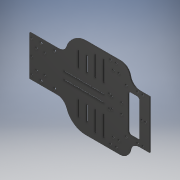
# Autodesk Inventor part: Base
Saved by Autodesk Inventor 2019 (Build 230136000, 136)
## iProperties
Created: 2019-07-29
Part Number: Base
Material: Résine phénolique
Document SubType Name: Modeling
Designer: Sébastien DI MERCURIO
Mass: 119.758 g
Surface Area: 806.74 cm^2
Volume: 86.7812 cm^3
Density: 1.38 g/cm^3
Appearance: Lisse - Noir
Author: Sébastien DI MERCURIO
Autodesk Inventor part; units mm, degrees
ref_plane "YZ Plane" through (0, 0, 0) normal (1, 0, 0) x (0, 1, 0)
ref_plane "XZ Plane" through (0, 0, 0) normal (0, 1, 0) x (-1, 0, 0)
ref_plane "XY Plane" through (0, 0, 0) normal (0, 0, 1) x (1, 0, 0)
sketch "Esquisse1" plane through (0, 0, 0) normal (0, 0, 1) x (1, 0, 0)
  line L0 (-242, 163) -> (0, 163)
  line L1 (0, 163) -> (0, 0)
  line L2 (0, 0) -> (-242, 0)
  line L3 (-242, 0) -> (-242, 163)
  dimension "d0" = 242
  dimension "d1" = 163
  constraints: 8 end point, 2 parallel, 1 horizontal, 1 perpendicular
  measures "d0" distance of L0.start L0.end
  measures "d1" distance of L0.end L1.end
extrude "Extrusion1" add sketch "Esquisse1" along normal blind 2.2
sketch "Esquisse2" plane through (0, 0, 2.2) normal (0, 0, 1) x (1, 0, 0)
  line L0 (0, 0) -> (-40, 0)
  line L1 (-40, 0) -> (-40, 33)
  line L2 (-40, 33) -> (0, 33)
  line L3 (0, 33) -> (0, 0)
  line L4 (0, 163) -> (-242, 163) projected
  line L5 (0, 163) -> (-40, 163)
  line L6 (-40, 163) -> (-40, 130)
  line L7 (-40, 130) -> (0, 130)
  line L8 (0, 130) -> (0, 163)
  line L9 (-242, 163) -> (-166, 163)
  line L10 (-166, 163) -> (-166, 121.5)
  line L11 (-166, 121.5) -> (-242, 121.5)
  line L12 (-242, 121.5) -> (-242, 163)
  line L13 (-242, 0) -> (-166, 0)
  line L14 (-166, 0) -> (-166, 41.5)
  line L15 (-166, 41.5) -> (-242, 41.5)
  line L16 (-242, 41.5) -> (-242, 0)
  dimension "d4" = 97
  dimension "d5" = 80
  dimension "d6" = 76
  dimension "d7" = 40
  constraints: 32 end point, 8 parallel, 4 horizontal, 4 perpendicular, 4 point on line, 2 collinear
  measures "d4" distance of L2.end L7.end
  measures "d5" distance between parallel lines of L15 L11
  measures "d6" distance of L14.end L15.end
  measures "d7" distance of L1.end L2.end
extrude "Extrusion2" cut sketch "Esquisse2" against normal through all
sketch "Esquisse3" plane through (0, 0, 2.2) normal (0, 0, 1) x (1, 0, 0)
  line L0 (-43, 119.5) -> (-20, 119.5)
  line L1 (-20, 119.5) -> (-20, 43.5)
  line L2 (-20, 43.5) -> (-43, 43.5)
  line L3 (-43, 43.5) -> (-43, 119.5)
  line L4 (0, 33) -> (0, 130) projected
  line L5 (0, 130) -> (-40, 130) projected
  line L6 (-92, 149.5) -> (-92, 109.5) construction
  line L7 (-93.5, 149.5) -> (-93.5, 109.5)
  line L8 (-90.5, 109.5) -> (-90.5, 149.5)
  arc A0 (-90.5, 149.5) -> (-93.5, 149.5) centre (-92, 149.5) ccw
  arc A1 (-93.5, 109.5) -> (-90.5, 109.5) centre (-92, 109.5) ccw
  line L9 (-109, 149.5) -> (-109, 109.5) construction
  line L10 (-110.5, 149.5) -> (-110.5, 109.5)
  line L11 (-107.5, 109.5) -> (-107.5, 149.5)
  arc A2 (-107.5, 149.5) -> (-110.5, 149.5) centre (-109, 149.5) ccw
  arc A3 (-110.5, 109.5) -> (-107.5, 109.5) centre (-109, 109.5) ccw
  line L12 (-126, 139.5) -> (-126, 109.5) construction
  line L13 (-127.5, 139.5) -> (-127.5, 109.5)
  line L14 (-124.5, 109.5) -> (-124.5, 139.5)
  arc A4 (-124.5, 139.5) -> (-127.5, 139.5) centre (-126, 139.5) ccw
  arc A5 (-127.5, 109.5) -> (-124.5, 109.5) centre (-126, 109.5) ccw
  line L15 (-143, 139.5) -> (-143, 109.5) construction
  line L16 (-144.5, 139.5) -> (-144.5, 109.5)
  line L17 (-141.5, 109.5) -> (-141.5, 139.5)
  arc A6 (-141.5, 139.5) -> (-144.5, 139.5) centre (-143, 139.5) ccw
  arc A7 (-144.5, 109.5) -> (-141.5, 109.5) centre (-143, 109.5) ccw
  line L18 (-172, 89) -> (-92, 89) construction
  line L19 (-172, 90.5) -> (-92, 90.5)
  line L20 (-92, 87.5) -> (-172, 87.5)
  arc A8 (-172, 90.5) -> (-172, 87.5) centre (-172, 89) ccw
  arc A9 (-92, 87.5) -> (-92, 90.5) centre (-92, 89) ccw
  line L21 (-172, 74) -> (-92, 74) construction
  line L22 (-172, 72.5) -> (-92, 72.5)
  line L23 (-92, 75.5) -> (-172, 75.5)
  arc A10 (-172, 75.5) -> (-172, 72.5) centre (-172, 74) ccw
  arc A11 (-92, 72.5) -> (-92, 75.5) centre (-92, 74) ccw
  line L24 (-92, 53.5) -> (-92, 13.5) construction
  line L25 (-93.5, 53.5) -> (-93.5, 13.5)
  line L26 (-90.5, 13.5) -> (-90.5, 53.5)
  arc A12 (-90.5, 53.5) -> (-93.5, 53.5) centre (-92, 53.5) ccw
  arc A13 (-93.5, 13.5) -> (-90.5, 13.5) centre (-92, 13.5) ccw
  line L27 (-109, 53.5) -> (-109, 13.5) construction
  line L28 (-110.5, 53.5) -> (-110.5, 13.5)
  line L29 (-107.5, 13.5) -> (-107.5, 53.5)
  arc A14 (-107.5, 53.5) -> (-110.5, 53.5) centre (-109, 53.5) ccw
  arc A15 (-110.5, 13.5) -> (-107.5, 13.5) centre (-109, 13.5) ccw
  line L30 (-126, 53.5) -> (-126, 23.5) construction
  line L31 (-127.5, 53.5) -> (-127.5, 23.5)
  line L32 (-124.5, 23.5) -> (-124.5, 53.5)
  arc A16 (-124.5, 53.5) -> (-127.5, 53.5) centre (-126, 53.5) ccw
  arc A17 (-127.5, 23.5) -> (-124.5, 23.5) centre (-126, 23.5) ccw
  line L33 (-143, 53.5) -> (-143, 23.5) construction
  line L34 (-144.5, 53.5) -> (-144.5, 23.5)
  line L35 (-141.5, 23.5) -> (-141.5, 53.5)
  arc A18 (-141.5, 53.5) -> (-144.5, 53.5) centre (-143, 53.5) ccw
  arc A19 (-144.5, 23.5) -> (-141.5, 23.5) centre (-143, 23.5) ccw
  line L36 (-246.6033, 81.5) -> (11.7947, 81.5)
  point P0 (0, 0)
  point P1 (-92, 129.5)
  point P2 (-109, 129.5)
  point P3 (-126, 124.5)
  point P4 (-143, 124.5)
  point P5 (-132, 89)
  point P6 (-132, 74)
  point P7 (-92, 33.5)
  point P8 (-109, 33.5)
  point P9 (-126, 38.5)
  point P10 (-143, 38.5)
  point P11 (-90.5, 89)
  dimension "d10" = 23
  dimension "d11" = 76
  dimension "d12" = 20
  dimension "d14" = 97
  dimension "d15" = 10.5
  dimension "d16" = 3
  dimension "d17" = 3
  dimension "d18" = 3
  dimension "d19" = 3
  dimension "d20" = 3
  dimension "d21" = 3
  dimension "d22" = 3
  dimension "d23" = 3
  dimension "d24" = 3
  dimension "d25" = 3
  dimension "d26" = 12
  dimension "d27" = 14
  dimension "d28" = 14
  dimension "d29" = 14
  dimension "d30" = 33
  dimension "d32" = 43
  dimension "d33" = 80
  dimension "d34" = 92
  dimension "d35" = 48.5
  dimension "d36" = 6
  dimension "d37" = 19
  dimension "d38" = 19
  constraints: 90 end point, 41 point on circle, 40 tangent, 20 centre point, 17 parallel, 10 midpoint, 8 point on line, 7 equal length, 6 horizontal alignment, 2 horizontal, 2 perpendicular, 2 vertical alignment, 1 vertical
  measures "d10" distance of L1.end L2.end
  measures "d11" distance of L0.end L1.end
  measures "d12" distance between parallel lines of L4 L1
  measures "d14" distance of L4.start L4.end
  measures "d15" distance between parallel lines of L0 L5
  measures "d16" distance between parallel lines of L17 L16
  measures "d17" distance between parallel lines of L35 L34
  measures "d18" distance between parallel lines of L32 L31
  measures "d19" distance between parallel lines of L14 L13
  measures "d20" distance between parallel lines of L11 L10
  measures "d21" distance between parallel lines of L8 L7
  measures "d22" distance between parallel lines of L29 L28
  measures "d23" distance between parallel lines of L26 L25
  measures "d24" distance between parallel lines of L20 L19
  measures "d25" distance between parallel lines of L22 L23
  measures "d26" distance between parallel lines of L23 L20
  measures "d27" distance between parallel lines of L7 L11
  measures "d28" distance between parallel lines of L10 L14
  measures "d29" distance between parallel lines of L13 L17
  measures "d33" distance of L18.end L18.start
  measures "d34" distance from line of L18.end L4
  measures "d35" distance between parallel lines of L5 L36
  measures "d36" distance between parallel lines of L36 L20
  measures "d37" distance from line of L19 L6.end
  measures "d38" distance from line of L22 L24.start
extrude "Extrusion3" cut sketch "Esquisse3" against normal through all
sketch "Esquisse4" plane through (0, 0, 2.2) normal (0, 0, 1) x (1, 0, 0)
  line L0 (-257.905, 81.5) -> (33.7686, 81.5)
  line L1 (-40, 33) -> (0, 33) construction
  line L2 (0, 130) -> (-40, 130) construction
  circle A0 centre (-15, 81.5) radius 1.5
  circle A1 centre (-8, 81.5) radius 1.5
  circle A2 centre (-13, 126.5) radius 1.5
  circle A3 centre (-24, 126.5) radius 1.5
  circle A4 centre (-47, 126.5) radius 1.5
  circle A5 centre (-67, 155) radius 1.5
  circle A6 centre (-78.5, 155) radius 1.5
  circle A7 centre (-73, 140) radius 1.5
  circle A8 centre (-61.5, 140) radius 1.5
  circle A9 centre (-56, 91.5) radius 1.5
  circle A10 centre (-76, 92.5) radius 1.5
  circle A11 centre (-81, 94.5) radius 1.5
  circle A12 centre (-228, 101) radius 1.5
  circle A13 centre (-211, 101) radius 1.5
  circle A14 centre (-237.5, 113.5) radius 1.5
  circle A15 centre (-237.5, 81.5) radius 1.5
  circle A16 centre (-218.5, 114.5) radius 2
  circle A17 centre (-191, 114.5) radius 2
  circle A18 centre (-218.5, 48.5) radius 2
  circle A19 centre (-228, 62) radius 1.5
  circle A20 centre (-211, 62) radius 1.5
  circle A21 centre (-237.5, 49.5) radius 1.5
  circle A22 centre (-191, 48.5) radius 2
  circle A23 centre (-13, 36.5) radius 1.5
  circle A24 centre (-24, 36.5) radius 1.5
  circle A25 centre (-47, 36.5) radius 1.5
  circle A26 centre (-67, 8) radius 1.5
  circle A27 centre (-78.5, 8) radius 1.5
  circle A28 centre (-73, 23) radius 1.5
  circle A29 centre (-61.5, 23) radius 1.5
  circle A30 centre (-56, 71.5) radius 1.5
  circle A31 centre (-76, 70.5) radius 1.5
  circle A32 centre (-81, 68.5) radius 1.5
  line L3 (-166, 121.5) -> (-242, 121.5) construction
  line L4 (-242, 121.5) -> (-242, 41.5) construction
  line L5 (-20, 119.5) -> (-20, 43.5) construction
  line L6 (0, 33) -> (0, 130) construction
  line L7 (-43, 43.5) -> (-43, 119.5) construction
  point P0 (0, 0)
  dimension "d41" = 97
  dimension "d42" = 48.5
  dimension "d43" = 3
  dimension "d44" = 4
  dimension "d46" = 7
  dimension "d47" = 7
  dimension "d48" = 27.5
  dimension "d49" = 23.5
  dimension "d50" = 32
  dimension "d51" = 4.5
  dimension "d52" = 4.5
  dimension "d53" = 20.5
  dimension "d54" = 20.5
  dimension "d55" = 17
  dimension "d56" = 14
  dimension "d57" = 7
  dimension "d59" = 13
  dimension "d60" = 11
  dimension "d61" = 23
  dimension "d62" = 3.5
  dimension "d63" = 3.5
  dimension "d64" = 3.5
  dimension "d65" = 20
  dimension "d66" = 22
  dimension "d67" = 26
  dimension "d68" = 13
  dimension "d69" = 33
  dimension "d70" = 38
  dimension "d71" = 117
  dimension "d72" = 147
  dimension "d73" = 147
  dimension "d74" = 117
  dimension "d75" = 11.5
  dimension "d76" = 11.5
  dimension "d77" = 61.5
  dimension "d78" = 67
  dimension "d91" = 8
  constraints: 33 centre point, 16 equal radius, 15 symmetric about line, 3 point on line, 2 end point, 1 horizontal, 15 other
  measures "d41" distance between parallel lines of L1 L2
  measures "d42" distance between parallel lines of L2 L0
  measures "d43" diameter of A6
  measures "d44" diameter of A16
  measures "d46" distance from line of L3 A17.centre
  measures "d47" distance from line of L3 A16.centre
  measures "d48" distance of A17.centre A16.centre
  measures "d49" distance from line of L4 A16.centre
  measures "d50" distance of A15.centre A14.centre
  measures "d51" distance from line of L4 A14.centre
  measures "d52" distance from line of L4 A15.centre
  measures "d53" distance from line of L3 A12.centre
  measures "d54" distance from line of L3 A13.centre
  measures "d55" distance of A13.centre A12.centre
  measures "d56" distance from line of L4 A12.centre
  measures "d57" distance of A1.centre A0.centre
  measures "d59" distance from line of L6 A2.centre
  measures "d60" distance of A2.centre A3.centre
  measures "d61" distance of A3.centre A4.centre
  measures "d62" distance from line of L2 A2.centre
  measures "d63" distance from line of L2 A3.centre
  measures "d64" distance from line of L2 A4.centre
  measures "d65" distance of A30.centre A9.centre
  measures "d66" distance of A31.centre A10.centre
  measures "d67" distance of A32.centre A11.centre
  measures "d68" distance from line of A9.centre L7
  measures "d69" distance from line of L7 A10.centre
  measures "d70" distance from line of L7 A11.centre
  measures "d71" distance of A29.centre A8.centre
  measures "d72" distance of A26.centre A5.centre
  measures "d73" distance of A6.centre A27.centre
  measures "d74" distance of A7.centre A28.centre
  measures "d75" distance of A8.centre A7.centre
  measures "d76" distance of A5.centre A6.centre
  measures "d77" distance from line of L6 A8.centre
  measures "d78" distance from line of L6 A5.centre
  measures "d91" distance from line of L6 A1.centre
extrude "Extrusion4" cut sketch "Esquisse4" against normal through all
chamfer "Chanfrein1" distance 1.5 angle 45 29 edges at (-239, 113.5, 2.2) (-229.5, 101, 2.2) (-212.5, 101, 2.2) (-239, 81.5, 2.2) (-229.5, 62, 2.2) (-212.5, 62, 2.2) (-239, 49.5, 2.2) (-82.5, 94.5, 2.2) (-77.5, 92.5, 2.2) (-57.5, 91.5, 2.2) (-77.5, 70.5, 2.2) (-82.5, 68.5, 2.2) (-57.5, 71.5, 2.2) (-16.5, 81.5, 2.2) (-9.5, 81.5, 2.2) (-14.5, 126.5, 2.2) (-25.5, 126.5, 2.2) (-48.5, 126.5, 2.2) (-63, 140, 2.2) (-74.5, 140, 2.2) (-80, 155, 2.2) (-68.5, 155, 2.2) (-74.5, 23, 2.2) (-63, 23, 2.2) (-68.5, 8, 2.2) (-80, 8, 2.2) (-48.5, 36.5, 2.2) (-25.5, 36.5, 2.2) (-14.5, 36.5, 2.2)
chamfer "Chanfrein2" distance 1.5 angle 45 4 edges at (-220.5, 48.5, 2.2) (-193, 48.5, 2.2) (-220.5, 114.5, 2.2) (-193, 114.5, 2.2)
fillet "Congé1" radius 5 4 edges at (-20, 119.5, 1.1) (-43, 119.5, 1.1) (-20, 43.5, 1.1) (-43, 43.5, 1.1)
fillet "Congé2" radius 20 4 edges at (-40, 130, 1.1) (-40, 33, 1.1) (-166, 41.5, 1.1) (-166, 121.5, 1.1)
fillet "Congé3" radius 20 2 edges at (-40, 163, 1.1) (-40, 0, 1.1)
fillet "Congé4" radius 40 2 edges at (-166, 163, 1.1) (-166, 0, 1.1)
equation "\"d15\" = -0.5 * d11 + 0.5 * d14"
equation "\"d17\" = d16"
equation "\"d18\" = d16"
equation "\"d19\" = d16"
equation "\"d20\" = d16"
equation "\"d21\" = d16"
equation "\"d22\" = d16"
equation "\"d23\" = d16"
equation "\"d24\" = d16"
equation "\"d25\" = d16"
equation "\"d35\" = 0.5 * d14"
equation "\"d36\" = 0.5 * d26"
equation "\"d38\" = d37"
equation "\"d42\" = 0.5 * d41"
equation "\"d47\" = d46"
equation "\"d52\" = d51"
equation "\"d54\" = d53"
equation "\"d63\" = d62"
equation "\"d64\" = d62"
equation "\"d73\" = d72"
equation "\"d74\" = d71"
equation "\"d76\" = d75"
